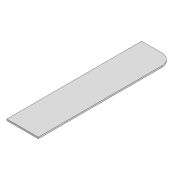
# Autodesk Inventor part: sidewall inside
Saved by Autodesk Inventor 2020 (Build 240168000, 168)
## iProperties
Created: 2020-03-01
Part Number: sidewall inside
Material: Generic
Document SubType Name: Modeling
Designer: ball
Density: 1 g/cm^3
Appearance: Default
Author: ball
Autodesk Inventor part; units mm, degrees
ref_plane "YZ Plane" through (0, 0, 0) normal (1, 0, 0) x (0, 1, 0)
ref_plane "XZ Plane" through (0, 0, 0) normal (0, 1, 0) x (-1, 0, 0)
ref_plane "XY Plane" through (0, 0, 0) normal (0, 0, 1) x (1, 0, 0)
sketch "Sketch1" plane through (0, 0, 0) normal (0, 1, 0) x (-1, 0, 0)
  line L0 (0, 0) -> (104.9602, 0)
  line L1 (104.9602, 0) -> (104.9602, -450.85)
  line L2 (104.9602, -450.85) -> (38.1, -450.85)
  line L3 (0, -412.75) -> (0, 0)
  arc A0 (0, -412.75) -> (38.1, -450.85) centre (38.1, -412.75) ccw
  line L4 (38.1, -412.75) -> (38.1, -450.85) construction
  line L5 (38.1, -412.75) -> (76.2, -412.75) construction
  dimension "d1" = 450.85
  dimension "d5" = 38.1
  dimension "d6" = 90
  dimension "d7" = 104.9602
  dimension "d8" = 38.1
  constraints: 12 end point, 2 horizontal, 2 parallel, 2 perpendicular, 2 point on circle, 1 centre point, 1 coincident
  measures "d1" distance of L0.end L1.end
  measures "d5" radius of A0
  measures "d6" angle of L4 L5
  measures "d7" distance between parallel lines of L3 L1
  measures "d8" distance from line of L3 point (38.1, -412.75)
extrude "Extrusion1" add sketch "Sketch1" along normal blind 5
body "Solid1"
